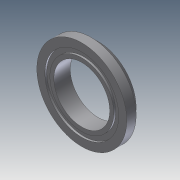
# Autodesk Inventor part: KMB1201T 機械油封
Saved by Autodesk Inventor 2012 SP2 (Build 160219200, 219)
## iProperties
Created: 2015-05-18
Part Number: KMB1201T 機械油封
Material: Default
Document SubType Name: Modeling
Designer: ERIC
Density: 1 g/cm^3
Author: ERIC
Autodesk Inventor part; units mm, degrees
ref_plane "YZ Plane" through (0, 0, 0) normal (1, 0, 0) x (0, 1, 0)
ref_plane "XZ Plane" through (0, 0, 0) normal (0, 1, 0) x (-1, 0, 0)
ref_plane "XY Plane" through (0, 0, 0) normal (0, 0, 1) x (1, 0, 0)
sketch "草圖1" plane through (0, 0, 0) normal (0, 0, 1) x (1, 0, 0)
  line L0 (0, 0) -> (0, 8.2)
  line L1 (0, 0) -> (22.5, 0)
  line L2 (0, 8.2) -> (19, 8.2)
  line L3 (22.5, 0) -> (22.5, 4.7)
  line L4 (22.5, 4.7) -> (19, 8.2)
  line L5 (14, 8.2) -> (14, 0)
  line L6 (16, 0) -> (18.5, 0)
  line L7 (18.5, 0) -> (18.5, 1)
  line L8 (18.5, 1) -> (16, 1)
  line L9 (16, 1) -> (16, 0)
  dimension "d1" = 8.2
  dimension "d2" = 45
  dimension "d3" = 38
  dimension "d5" = 135
  dimension "d6" = 28
  dimension "d7" = 32
  dimension "d8" = 37
  dimension "d9" = 1
  constraints: 20 end point, 4 perpendicular, 3 parallel, 3 point on line, 1 horizontal, 1 vertical
  measures "d1" distance of L0.start L0.end
  measures "d2" diameter of L1.end L0
  measures "d3" diameter of L2.end L0
  measures "d5" angle of L4 L2
  measures "d6" diameter of L5 L0
  measures "d7" diameter of L9 L0
  measures "d8" diameter of L7 L0
  measures "d9" distance of L6.end L7.end
revolve "迴轉1" add sketch "草圖1" angle 360 about axis through (0, 0, 0) along (0, 1, 0) contours L5 L2 L4 L3 L1 L7 L8 L9
